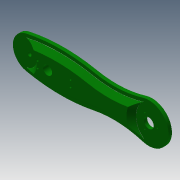
# Autodesk Inventor part: rameno(b)dole
Saved by Autodesk Inventor 2013 (Build 170138000, 138)
## iProperties
Created: 2013-05-25
Part Number: rameno(b)dole
Material: Generic
Document SubType Name: Modeling
Designer: idle-rug
Density: 1 g/cm^3
Author: idle-rug
Autodesk Inventor part; units mm, degrees
ref_plane "YZ Plane" through (0, 0, 0) normal (1, 0, 0) x (0, 1, 0)
ref_plane "XZ Plane" through (0, 0, 0) normal (0, 1, 0) x (-1, 0, 0)
ref_plane "XY Plane" through (0, 0, 0) normal (0, 0, 1) x (1, 0, 0)
sketch "Sketch1" plane through (0, 0, 0) normal (0, 1, 0) x (-1, 0, 0)
  line L0 (-90, -25) -> (90, -25)
  line L1 (90, -25) -> (90, 25)
  line L2 (90, 25) -> (-90, 25)
  line L3 (-90, 25) -> (-90, -25)
  line L4 (-90, -25) -> (90, 25) construction
  line L5 (90, -25) -> (-90, 25) construction
  circle A0 centre (90, 0) radius 25
  circle A1 centre (-90, 0) radius 25
  point P0 (0, 0)
  dimension "d0" = 180
  dimension "d1" = 50
  constraints: 12 end point, 4 midpoint, 2 parallel, 2 vertical alignment, 1 horizontal, 1 perpendicular, 4 other
  measures "d0" distance of L2.end L1.end
  measures "d1" distance of L1.end L0.end
extrude "Extrusion1" add sketch "Sketch1" along normal blind 5
sketch "Sketch2" plane through (0, 5, 0) normal (0, 1, 0) x (1, 0, 0)
  arc A0 (90, -25) -> (90, 25) centre (90, 0) ccw projected
  arc A1 (-90, 25) -> (-90, -25) centre (-90, 0) ccw projected
  circle A2 centre (-90, 0) radius 7.5
  circle A3 centre (90, 0) radius 7.5
  point P0 (0, 0)
  dimension "d4" = 15
  dimension "d5" = 15
  constraints: 2 centre point, 2 coincident
  measures "d4" diameter of A2
  measures "d5" diameter of A3
extrude "Extrusion2" cut sketch "Sketch2" against normal blind 5
sketch "Sketch3" plane through (0, 0, 0) normal (0, -1, 0) x (1, 0, 0)
  line L0 (-90, 25) -> (90, 25) projected
  arc A0 (-90, 25) -> (-90, -25) centre (-90, 0) ccw projected
  line L1 (-90, 0) -> (-55.35, 0)
  circle A1 centre (-55.35, 0) radius 17.325
  line L2 (-55.35, 0) -> (-73.45, 0)
  line L3 (-73.45, 0) -> (-18.45, 0)
  line L4 (-18.45, 10) -> (-73.45, 10)
  line L5 (-73.45, 10) -> (-73.45, -10)
  line L6 (-73.45, -10) -> (-18.45, -10)
  line L7 (-18.45, -10) -> (-18.45, 10)
  line L8 (-18.45, 10) -> (-73.45, -10) construction
  line L9 (-73.45, 10) -> (-18.45, -10) construction
  line L10 (-25.85, -10) -> (-25.85, 10)
  line L11 (-25.85, 10) -> (-66.05, -10) construction
  line L12 (-66.05, 10) -> (-25.85, -10) construction
  line L13 (-70.8, 4.95) -> (-70.8, -4.95)
  line L14 (-70.8, -4.95) -> (-61.3, -4.95)
  line L15 (-61.3, -4.95) -> (-61.3, 4.95)
  line L16 (-61.3, 4.95) -> (-70.8, -4.95) construction
  line L17 (-70.8, 4.95) -> (-61.3, -4.95) construction
  line L18 (-21.1, 4.95) -> (-30.6, 4.95)
  line L19 (-30.6, 4.95) -> (-30.6, -4.95)
  line L20 (-30.6, -4.95) -> (-21.1, -4.95)
  line L21 (-21.1, -4.95) -> (-21.1, 4.95)
  line L22 (-21.1, 4.95) -> (-30.6, -4.95) construction
  line L23 (-30.6, 4.95) -> (-21.1, -4.95) construction
  circle A2 centre (-70.8, 4.95) radius 1.5
  circle A3 centre (-70.8, -4.95) radius 1.5
  circle A4 centre (-21.1, -4.95) radius 1.5
  circle A5 centre (-21.1, 4.95) radius 1.5
  circle A6 centre (-55.35, 0) radius 6.8
  point P0 (0, 0)
  point P1 (-45.95, 0)
  point P2 (-45.95, 0)
  point P3 (-66.05, 0)
  point P4 (-25.85, 0)
  dimension "d9" = 34.65
  dimension "d10" = 18.1
  dimension "d11" = 55
  dimension "d12" = 20
  dimension "d13" = 40.2
  dimension "d14" = 9.5
  dimension "d15" = 9.9
  dimension "d16" = 9.5
  dimension "d17" = 9.9
  dimension "d18" = 3
  dimension "d19" = 3
  dimension "d20" = 3
  dimension "d21" = 3
  dimension "d22" = 13.6
  constraints: 46 end point, 11 midpoint, 7 coincident, 6 centre point, 6 parallel, 3 point on line, 2 horizontal, 2 perpendicular
  measures "d9" distance of L1.start L1.end
  measures "d10" distance of L2.start L2.end
  measures "d11" distance of L2.end L3.end
  measures "d12" distance of L5.end L4.end
  measures "d13" distance of L10.start L11.end
  measures "d14" distance of L14.end L13.end
  measures "d15" distance of L13.end L13.start
  measures "d16" distance of L20.end L19.end
  measures "d17" distance of L19.end L18.end
  measures "d18" diameter of A2
  measures "d19" diameter of A3
  measures "d20" diameter of A4
  measures "d21" diameter of A5
  measures "d22" diameter of A6
extrude "Extrusion3" cut sketch "Sketch3" against normal blind 5 contours A2 A1 | A1 A2 | A3 L13 L14 A1 | A1 A3 | A6 L15 L1 | L1 L15 A6 | A3 L14 L13 | L15 A6 L3 L1 | L1 L3 A6 L15 | A5 L21 L18 | L18 L21 A5 | A4 L21 L20 | L20 L21 A4
sketch "Sketch4" plane through (0, 0, 0) normal (0, -1, 0) x (1, 0, 0)
  circle A0 centre (90, 0) radius 7.5 projected
  arc A1 (90, -25) -> (90, 25) centre (90, 0) ccw projected
  line L0 (-90, 25) -> (90, 25) projected
  circle A2 centre (90, 0) radius 17.5
  line L1 (82.5, 0) -> (72.5, 0)
  line L2 (97.5, 0) -> (107.5, 0)
  circle A3 centre (102.5, 0) radius 1
  line L3 (90, 0) -> (107.5, 0) construction
  line L4 (90, 0) -> (81.25, -15.1554)
  line L5 (90, 0) -> (107.5, 0) construction
  circle A4 centre (83.75, 10.8253) radius 1
  circle A5 centre (83.75, -10.8253) radius 1
  point P0 (0, 0)
  dimension "d26" = 2
  dimension "d29" = 2
  dimension "d30" = 2
  constraints: 10 end point, 5 point on circle, 4 centre point, 2 horizontal, 1 coincident, 1 collinear, 1 equal length, 1 midpoint, 1 parallel, 1 point on line
  measures "d26" diameter of A3
  measures "d29" diameter of A4
  measures "d30" diameter of A5
extrude "Extrusion4" cut sketch "Sketch4" against normal blind 5 contours A3 L2 | L2 A3 | A5 L4 | L4 A5 | A4
sketch "Sketch5" plane through (0, 0, 0) normal (0, -1, 0) x (1, 0, 0)
  circle A0 centre (83.75, 10.8253) radius 1 projected
  circle A1 centre (102.5, 0) radius 1 projected
  circle A2 centre (83.75, -10.8253) radius 1 projected
  circle A3 centre (-21.1, 4.95) radius 1.5 projected
  circle A4 centre (-70.8, -4.95) radius 1.5 projected
  circle A5 centre (-55.35, 0) radius 6.8 projected
  circle A6 centre (-70.8, 4.95) radius 1.5 projected
  circle A7 centre (-21.1, -4.95) radius 1.5 projected
  circle A8 centre (-90, 0) radius 7.5 projected
  circle A9 centre (90, 0) radius 7.5 projected
  line L0 (-55.35, 0) -> (0, 0)
  arc A10 (6.9815, 24.9874) -> (-95.2411, 24.4444) centre (-42.8301, -220) ccw
  arc A11 (6.9815, 24.9874) -> (81.1447, 28.6633) centre (36.8685, 171.9798) ccw
  line L1 (-115, 0) -> (115, 0)
  arc A12 (-95.2411, -24.4444) -> (6.9815, -24.9874) centre (-42.8301, 220) ccw
  arc A13 (81.1447, -28.6633) -> (6.9815, -24.9874) centre (36.8685, -171.9798) ccw
  arc A14 (-95.2411, 24.4444) -> (-95.2411, -24.4444) centre (-90, 0) ccw
  arc A15 (81.1447, -28.6633) -> (81.1447, 28.6633) centre (90, 0) ccw construction
  arc A16 (-95.2411, 24.4444) -> (-95.2411, -24.4444) centre (-90, 0) ccw
  arc A17 (81.1447, -28.6633) -> (81.1447, 28.6633) centre (90, 0) ccw
  constraints: 17 point on circle, 8 centre point, 5 symmetric about line, 5 tangent, 4 end point, 2 other
extrude "Extrusion5" add sketch "Sketch5" along normal blind 5
sketch "Sketch6" plane through (0, 5, 0) normal (0, 1, 0) x (1, 0, 0)
  circle A0 centre (83.75, -10.8253) radius 1 projected
  circle A1 centre (102.5, 0) radius 1 projected
  circle A2 centre (83.75, 10.8253) radius 1 projected
  circle A3 centre (-21.1, -4.95) radius 1.5 projected
  circle A4 centre (-70.8, 4.95) radius 1.5 projected
  circle A5 centre (-55.35, 0) radius 6.8 projected
  circle A6 centre (-70.8, -4.95) radius 1.5 projected
  circle A7 centre (-21.1, 4.95) radius 1.5 projected
  circle A8 centre (-90, 0) radius 7.5 projected
  circle A9 centre (90, 0) radius 7.5 projected
  line L0 (-90, -25) -> (90, -25) projected
  arc A10 (90, -25) -> (90, 25) centre (90, 0) ccw projected
  line L1 (90, 25) -> (-90, 25) projected
  arc A11 (-90, 25) -> (-90, -25) centre (-90, 0) ccw projected
  point P0 (0, 0)
extrude "Extrusion6" cut sketch "Sketch6" against normal blind 5
sketch "Sketch8" plane through (0, -5, 0) normal (0, -1, 0) x (1, 0, 0)
  circle A0 centre (-55.35, 0) radius 6.8 projected
  circle A1 centre (-21.1, -4.95) radius 1.5 projected
  circle A2 centre (-70.8, 4.95) radius 1.5 projected
  circle A3 centre (-70.8, -4.95) radius 1.5 projected
  circle A4 centre (-21.1, 4.95) radius 1.5 projected
  arc A5 (-95.2411, 24.4444) -> (-95.2411, -24.4444) centre (-90, 0) ccw projected
  arc A6 (81.1447, -28.6633) -> (81.1447, 28.6633) centre (90, 0) ccw projected
  arc A7 (5.9853, 20.0876) -> (-94.1929, 19.5556) centre (-42.8301, -220) ccw
  arc A8 (5.9853, 20.0876) -> (82.6206, 23.8861) centre (36.8685, 171.9798) ccw
  line L0 (-90, 0) -> (90, 0)
  arc A9 (-94.1929, -19.5556) -> (5.9853, -20.0876) centre (-42.8301, 220) ccw
  arc A10 (82.6206, -23.8861) -> (5.9853, -20.0876) centre (36.8685, -171.9798) ccw
  arc A11 (-94.1929, -19.5556) -> (-94.1929, 19.5556) centre (-98.3858, 0) ccw
  arc A12 (82.6206, 23.8861) -> (82.6206, -23.8861) centre (100.7715, 0) ccw
  point P0 (0, 0)
  dimension "d72" = 20
  dimension "d73" = 30
  constraints: 13 point on circle, 6 centre point, 5 symmetric about line, 2 coincident, 2 end point, 1 horizontal, 2 other
  measures "d72" radius of A11
  measures "d73" radius of A12
extrude "Extrusion7" add sketch "Sketch8" along normal blind 7.3 contours L0 A12 A10 A9 A11 A0 | A0 L0 A11 A7 A8 A12
sketch "Sketch14" plane through (0, 0, 0) normal (0, 1, 0) x (1, 0, 0)
  circle A0 centre (-90, 0) radius 7.5 projected
  arc A1 (-95.2411, 24.4444) -> (-95.2411, -24.4444) centre (-90, 0) ccw projected
  circle A2 centre (-90, 0) radius 3
  point P0 (0, 0)
  dimension "d103" = 6
  constraints: 1 centre point, 1 coincident
  measures "d103" diameter of A2
extrude "Extrusion13" add sketch "Sketch14" against normal blind 5
chamfer "Chamfer2" distance 7 angle 45 6 edges at (-44.1313, -12.3, 24.9965) (44.5417, -12.3, 17.1698) (70.7715, -12.3, 0) (44.5417, -12.3, -17.1698) (-44.1313, -12.3, -24.9965) (-78.3858, -12.3, 0)
body "Solid1"
